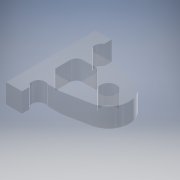
# Autodesk Inventor part: アームユニット底板締結パーツ3t用(4)
Saved by Autodesk Inventor 2020 (Build 240168000, 168)
## iProperties
Created: 2017-03-14
Part Number: アームユニット底板締結パーツ3t用(4)
Material: ポリカーボネート、クリア
Document SubType Name: Modeling
Designer: shiota
Mass: 0.288742 g
Surface Area: 3.73889 cm^2
Volume: 0.240619 cm^3
Density: 1.2 g/cm^3
Appearance: ポリカーボネート - クリア
Description: アルミ2000番.3t
Author: shiota
Autodesk Inventor part; units mm, degrees
ref_plane "YZ Plane" through (0, 0, 0) normal (1, 0, 0) x (0, 1, 0)
ref_plane "XZ Plane" through (0, 0, 0) normal (0, 1, 0) x (-1, 0, 0)
ref_plane "XY Plane" through (0, 0, 0) normal (0, 0, 1) x (1, 0, 0)
sketch "スケッチ1" plane through (0, 0, 0) normal (0, 0, 1) x (1, 0, 0)
  circle A0 centre (0, 0) radius 1.25
  arc A1 (0.6267, -3.189) -> (0.6267, 3.189) centre (0, 0) ccw
  line L0 (0, 0) -> (-4.5, 0)
  line L1 (-4.5, -4.1965) -> (-4.5, -4)
  line L2 (-4.5, 4) -> (-3.5, 4)
  line L3 (-3.5, 4) -> (0.6267, 3.189)
  line L4 (-4.5, -4) -> (-3.5, -4)
  line L5 (-3.5, -4) -> (0.6267, -3.189)
  line L6 (-4.5, 4) -> (-6.5, 4)
  line L7 (-4.5, -4) -> (-6.5, -4)
  line L8 (-9, 7) -> (-9, -7)
  line L9 (-9, -7) -> (-6.5, -7)
  line L10 (-9, 7) -> (-6.5, 7)
  line L11 (-6.5, 7) -> (-6.5, 4)
  line L12 (-6.5, -4) -> (-6.5, -7)
  dimension "d0" = 2.5
  dimension "d3" = 8
  dimension "d5" = 8
  dimension "d6" = 2
  dimension "d7" = 2
  dimension "d8" = 3
  dimension "d14" = 1
  dimension "d17" = 3
  dimension "d32" = 14
  dimension "d33" = 2.5
  dimension "d35" = 2
  constraints: 26 end point, 5 horizontal, 4 parallel, 4 perpendicular, 2 centre point, 2 coincident, 2 point on circle, 2 tangent, 2 vertical, 1 point on line
  measures "d0" diameter of A0
  measures "d3" distance of L2.end L4.end
  measures "d5" distance of L2.start L1.end
  measures "d6" distance of L2.start L6.end
  measures "d7" distance of L1.end L7.end
  measures "d8" distance from line of L6 L10.end
  measures "d14" distance of L1.end L4.end
  measures "d17" distance between parallel lines of L9 L7
  measures "d32" distance of L8.start L8.end
  measures "d33" distance of L8.end L9.end
  measures "d35" radial gap between concentric circles of A1 A0
extrude "押し出し1" add sketch "スケッチ1" along normal blind 3
sketch "スケッチ2" plane through (0, 0, 3) normal (0, 0, 1) x (1, 0, 0)
  line L0 (-6.5, 7) -> (-6.5, 4) projected
  circle A0 centre (-6, -4.9233) radius 1.05
  circle A1 centre (-6, 4.9233) radius 1.05
  point P0 (-4.5, 4)
  point P1 (-4.5, -4)
  dimension "d13" = 2.1
  dimension "d12" = 2.1
  dimension "d15" = 0.5
  constraints: 1 centre point, 3 other
  measures "d12" diameter of A0
  measures "d15" distance from line of L0 point (-6, 4.923)
extrude "押し出し2" cut sketch "スケッチ2" against normal blind 3
sketch "スケッチ4" plane through (0, 0, 3) normal (0, 0, 1) x (1, 0, 0)
  line L0 (-9, -7) -> (-9, 7) projected
  line L1 (-3.5, -4) -> (-5.5, -4) projected
  line L2 (0.6267, -3.189) -> (-3.5, -4) projected
  line L3 (-3.5, 4) -> (0.6267, 3.189) projected
  line L4 (-5.5, 4) -> (-3.5, 4) projected
  circle A0 centre (0, 0) radius 1.25 projected
  line L5 (-7, 2) -> (-2.5617, 2)
  line L6 (-2.5617, -2) -> (-7, -2)
  line L7 (-7, -2) -> (-7, 2)
  arc A1 (-2.5617, 2) -> (-2.5617, -2) centre (0, 0) ccw
  arc A2 (0.6267, -3.189) -> (0.6267, 3.189) centre (0, 0) ccw
  dimension "d23" = 2
  dimension "d24" = 2
  dimension "d25" = 2
  constraints: 8 end point, 4 point on circle, 2 centre point, 1 coincident, 1 horizontal, 1 parallel
  measures "d23" distance between parallel lines of L5 L4
  measures "d24" distance between parallel lines of L1 L6
  measures "d25" distance between parallel lines of L0 L7
extrude "押し出し3" cut sketch "スケッチ4" against normal blind 3 contours L5 A1 L6 L7
fillet "フィレット1" radius 1 4 edges at (-2.5617, -2, 1.5) (-2.5617, 2, 1.5) (-7, -2, 1.5) (-7, 2, 1.5)
